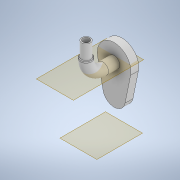
# Autodesk Inventor part: Vòi
Saved by Autodesk Inventor 2020 (Build 240168000, 168)
## iProperties
Created: 2022-09-22
Part Number: Vòi
Material: Generic
Document SubType Name: Modeling
Designer: ASUS
Density: 1 g/cm^3
Appearance: Default
Author: ASUS
Autodesk Inventor part; units mm, degrees
ref_plane "YZ Plane" through (0, 0, 0) normal (1, 0, 0) x (0, 1, 0)
ref_plane "XY Plane" through (0, 0, 0) normal (0, 0, 1) x (1, 0, 0)
sketch "Sketch1" plane through (0, 0, 0) normal (0, 0, 1) x (1, 0, 0)
  arc A0 (3.8578, 24.2337) -> (23.4537, 24.2337) centre (13.6558, 26.2337) ccw
  arc A1 (28.3527, 48.2337) -> (-1.0412, 48.2337) centre (13.6558, 51.2337) ccw
  line L0 (-1.0412, 48.2337) -> (3.8578, 24.2337)
  line L1 (28.3527, 48.2337) -> (23.4537, 24.2337)
  dimension "d32" = 20
  dimension "d33" = 30
  constraints: 5 tangent, 4 end point, 4 point on circle, 2 centre point
  measures "d32" diameter of A0
  measures "d33" diameter of A1
extrude "Extrusion8" add sketch "Sketch1" along normal blind 7
sketch "Sketch8" plane through (0, 0, 7) normal (0, 0, 1) x (1, 0, 0)
  arc A0 (28.3527, 48.2337) -> (-1.0412, 48.2337) centre (13.6558, 51.2337) ccw projected
  circle A1 centre (13.6558, 51.2337) radius 5
  point P0 (0, 0)
  dimension "d36" = 10
  constraints: 1 centre point, 1 coincident
  measures "d36" diameter of A1
extrude "Extrusion9" add sketch "Sketch8" along normal blind 40
ref_plane "Work Plane8" through (13.6558, 56.2337, 7) normal (0, 1, 0) x (-1, 0, 0)
sketch "Sketch13" plane through (0, 0, 0) normal (0, 0, -1) x (-1, 0, 0)
  circle A0 centre (-13.6558, 51.2337) radius 5 projected
  circle A1 centre (-13.6558, 51.2337) radius 5
  point P0 (0, 0)
  constraints: 1 centre point, 1 coincident
hole "Hole1" at (13.6558, 51.2337, 0) direction (0, 0, 1) diameter 6 end through all counterbore diameter 8 counterbore depth 7
sketch "Sketch14" plane through (13.6558, 51.2337, 47) normal (0, 0, 1) x (1, 0, 0)
  circle A0 centre (0, 0) radius 4
  arc A1 (14.6969, -3) -> (-14.6969, -3) centre (0, 0) ccw projected
  circle A2 centre (0, 0) radius 5
  point P0 (-13.6558, -51.2337)
  dimension "d52" = 8
  constraints: 2 centre point, 1 coincident
  measures "d52" diameter of A0
extrude "Extrusion11" cut sketch "Sketch14" against normal blind 13
sketch "Sketch15" plane through (13.6558, 56.2337, 7) normal (0, 1, 0) x (-1, 0, 0)
  line L0 (5, 10) -> (-5.1311, 10)
  line L1 (4, 40) -> (-4, 40) projected
  point P0 (13.6558, -7)
  dimension "d55" = 30
  constraints: 2 end point, 1 horizontal
  measures "d55" distance between parallel lines of L0 L1
bend part "Bend Part3" radius 10 angle 90 line through (8.6558, 56.2337, 17) along (1, 0, 0) centre toward (0, 1, 0) moving side (0, 0, 1) both sides no
body "Solid4"
